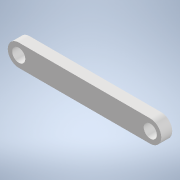
# Autodesk Inventor part: Part6
Saved by Autodesk Inventor 2022 (Build 260153000, 153)
## iProperties
Created: 2022-02-01
Part Number: Part6
Material: Generic
Document SubType Name: Modeling
Designer: br4ch
Density: 1 g/cm^3
Appearance: Default
Author: br4ch
Autodesk Inventor part; units mm, degrees
ref_plane "YZ Plane" through (0, 0, 0) normal (1, 0, 0) x (0, 1, 0)
ref_plane "XZ Plane" through (0, 0, 0) normal (0, 1, 0) x (-1, 0, 0)
ref_plane "XY Plane" through (0, 0, 0) normal (0, 0, 1) x (1, 0, 0)
sketch "Sketch1" plane through (0, 0, 0) normal (0, 0, 1) x (1, 0, 0)
  line L0 (-41, 14) -> (19, 14) construction
  line L1 (-41, 9) -> (19, 9)
  line L2 (19, 19) -> (-41, 19)
  arc A0 (-41, 19) -> (-41, 9) centre (-41, 14) ccw
  arc A1 (19, 9) -> (19, 19) centre (19, 14) ccw
  circle A2 centre (-41, 14) radius 3
  circle A3 centre (19, 14) radius 3
  point P0 (0, 0)
  point P1 (-11, 14)
  dimension "d0" = 10
  dimension "d1" = 6
  dimension "d3" = 60
  constraints: 8 end point, 4 centre point, 4 point on circle, 4 tangent, 2 coincident, 1 equal radius, 1 horizontal, 1 midpoint, 1 parallel
  measures "d0" diameter of A1
  measures "d1" diameter of A2
  measures "d3" distance of L0.end L0.start
extrude "Extrusion1" add sketch "Sketch1" along normal blind 5
equation "\"d0\" = R"
equation "\"d1\" = r"
equation "\"d4\" = th"
equation "\"th\" = 5"
equation "\"r\" = 6"
equation "\"R\" = 10"
body "Solid1"
